Autodesk Inventor part; units mm, degrees
(part 2 of 2)
  arc A313 (-1.0791, -115.8997) -> (-6.8196, -114.5524) centre (-4.0762, -115.7663) ccw construction
  line L219 (-36.7213, -133.8394) -> (-48.1249, -104.3532) construction
  arc A314 (-47.9204, -101.7631) -> (-48.1249, -104.3532) centre (-45.3269, -103.271) ccw construction
  arc A315 (-47.9204, -101.7631) -> (-47.8472, -101.6329) centre (-52.2429, -99.25) ccw construction
  arc A316 (-45.7421, -100.1103) -> (-47.8472, -101.6329) centre (-45.2099, -103.0627) ccw construction
  line L220 (-45.7421, -100.1103) -> (-41.234, -99.2976) construction
  arc A317 (-40.7018, -99.25) -> (-41.234, -99.2976) centre (-40.7018, -102.25) ccw construction
  line L221 (-40.7018, -99.25) -> (-12.8278, -99.25) construction
  arc A318 (-10.3603, -103.9563) -> (-12.8278, -99.25) centre (-12.8278, -102.25) ccw construction
  line L222 (-10.3603, -103.9563) -> (-31.4557, -134.4635) construction
  arc A319 (-36.7213, -133.8394) -> (-31.4557, -134.4635) centre (-33.9232, -132.7572) ccw construction
  line L223 (-20.8168, -202.1636) -> (-36.0643, -184.9732) construction
  arc A320 (-36.5634, -181.7686) -> (-36.0643, -184.9732) centre (-33.82, -182.9825) ccw construction
  line L224 (-36.5634, -181.7686) -> (-31.9746, -171.3986) construction
  arc A321 (-26.4332, -171.5305) -> (-31.9746, -171.3986) centre (-29.2312, -172.6126) ccw construction
  line L225 (-26.4332, -171.5305) -> (-15.7744, -199.0907) construction
  arc A322 (-20.8168, -202.1636) -> (-15.7744, -199.0907) centre (-18.5724, -200.1729) ccw construction
  spline S0 degree 3 poles (-317.2195, -95.25) (-317.2195, -95.1954) (-317.2285, -95.1401) (-317.273, -95.0007) (-317.3229, -94.9193) (-317.417, -94.8085) (-317.4554, -94.7708) (-317.4964, -94.7356) knots 0 0 0 0 0.273166 0.273166 0.731887 0.731887 1 1 1 1 construction
  line L226 (-317.2195, -307.25) -> (-317.2195, -95.25) construction
  spline S1 degree 3 poles (-317.4964, -307.7644) (-317.4545, -307.7284) (-317.4152, -307.6896) (-317.3423, -307.6031) (-317.3087, -307.5542) (-317.258, -307.4541) (-317.2397, -307.4032) (-317.2228, -307.3171) (-317.2195, -307.2834) (-317.2195, -307.25) knots 0 0 0 0 0.274359 0.274359 0.565441 0.565441 0.832862 0.832862 1 1 1 1 construction
  line L227 (-317.4964, -307.7644) -> (-317.4964, -308.25) construction
  line L228 (-317.4964, -308.25) -> (-367.8998, -308.25) construction
  arc A323 (-367.8998, -308.25) -> (-370.8998, -311.25) centre (-367.8998, -311.25) ccw construction
  line L229 (-370.8998, -311.25) -> (-408.6777, -397.2389) construction
  arc A324 (-408.6777, -397.2389) -> (-404.1, -404.25) centre (-404.1, -399.25) ccw construction
  line L230 (-404.1, -404.25) -> (6.1002, -404.25) construction
  arc A325 (6.1002, -404.25) -> (9.1002, -401.25) centre (6.1002, -401.25) ccw construction
  line L231 (9.1002, -401.25) -> (9.1002, -1.25) construction
  arc A326 (9.1002, -1.25) -> (6.1002, 1.75) centre (6.1002, -1.25) ccw construction
  line L232 (6.1002, 1.75) -> (-404.1, 1.75) construction
  arc A327 (-404.1, 1.75) -> (-408.6777, -5.2611) centre (-404.1, -3.25) ccw construction
  line L233 (-408.6777, -5.2611) -> (-370.8998, -91.25) construction
  arc A328 (-370.8998, -91.25) -> (-367.8998, -94.25) centre (-367.8998, -91.25) ccw construction
  line L234 (-367.8998, -94.25) -> (-317.4964, -94.25) construction
  line L235 (-317.4964, -94.25) -> (-317.4964, -94.7356) construction
  arc A329 (-3, -2) -> (9, -2) centre (3, -2) ccw construction
  line L236 (6, -2) -> (9, -2) construction
  line L237 (6, 0) -> (6, -2) construction
  line L238 (0, 0) -> (6, 0) construction
  line L239 (0, -2) -> (0, 0) construction
  line L240 (-3, -2) -> (0, -2) construction
  circle A330 centre (3, -2.65) radius 2.625 construction
  line L241 (4.1002, -9.25) -> (4.1002, -53.25)
  arc A331 (4.1002, -9.25) -> (1.1002, -6.25) centre (1.1002, -9.25) ccw
  arc A332 (-3, -2) -> (9, -2) centre (3, -2) ccw
  line L242 (-155.8998, -6.25) -> (1.1002, -6.25)
  point P0 (3, 0)
  point P1 (-1.2353, -6.25)
  point P2 (3.802, -7.9462)
extrude "Выдавливание4" cut sketch "Эскиз4" against normal blind 6
fillet "Сопряжение2" radius 2 2 edges at (-4.5, -8.25, 2) (4.5, -8.25, 2)
chamfer "Фаска2" distance 2 angle 45 1 edges at (0, -4.25, 2)
fillet "Сопряжение3" radius 6 2 edges at (-6, 6, 1) (6, 6, 1)
equation "\"d18\" = d16"
